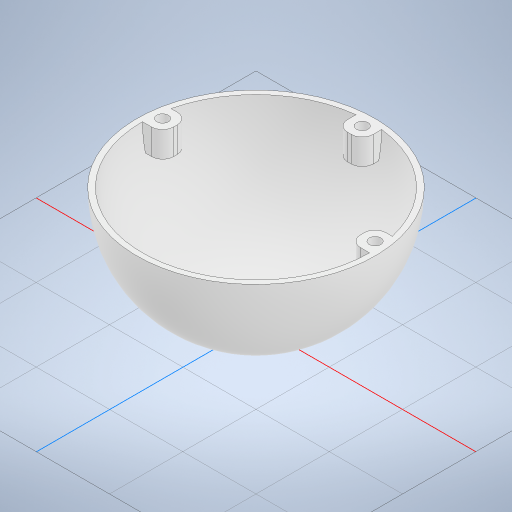
# Autodesk Inventor part: Kugel_part1_halbkugel
Saved by Autodesk Inventor 2023 (Build 270158000, 158)
## iProperties
Created: 2022-07-05
Part Number: Kugel_part1_halbkugel
Material: FormLabs Resin
Document SubType Name: Modeling
Designer: dennis
Density: 1.06 g/cm^3
Appearance: Smooth - White
Author: dennis
Autodesk Inventor part; units mm, degrees
ref_plane "YZ Plane" through (0, 0, 0) normal (1, 0, 0) x (0, 1, 0)
ref_plane "XZ Plane" through (0, 0, 0) normal (0, 1, 0) x (-1, 0, 0)
ref_plane "XY Plane" through (0, 0, 0) normal (0, 0, 1) x (1, 0, 0)
sketch "Skizze1" plane through (0, 0, 0) normal (0, 1, 0) x (-1, 0, 0)
  arc A0 (-32.5, 0) -> (32.5, 0) centre (0, 0) ccw
  line L0 (32.5, 0) -> (-32.5, 0)
  circle A1 centre (0, 0) radius 32.5
  line L1 (32.5, 0) -> (25.5, 0)
  line L2 (25.5, 0) -> (25.5, -7)
  line L3 (25.5, -7) -> (32.5, -7)
  line L4 (32.5, -7) -> (32.5, 0)
  line L5 (-32.5, 0) -> (-25.5, 0)
  line L6 (-25.5, 0) -> (-25.5, -7)
  line L7 (-25.5, -7) -> (-32.5, -7)
  line L8 (-32.5, -7) -> (-32.5, 0)
  line L9 (-3.5, -25.5) -> (3.5, -25.5)
  line L10 (3.5, -25.5) -> (3.5, -32.5)
  line L11 (3.5, -32.5) -> (-3.5, -32.5)
  line L12 (-3.5, -32.5) -> (-3.5, -25.5)
  line L13 (0, 0) -> (0, -32.5)
  circle A2 centre (29, -3.5) radius 1.6
  circle A3 centre (-29, -3.5) radius 1.6
  circle A4 centre (0, -29) radius 1.6
  point P0 (32.5, 0)
  point P1 (-31.7372, -7)
  point P2 (-25.5, 0)
  point P3 (-3.5, -32.311)
  point P4 (3.5, -32.311)
  point P5 (31.7372, -7)
  dimension "d0" = 65
  dimension "d2" = 65
  dimension "d3" = 7
  dimension "d4" = 7
  dimension "d5" = 7
  dimension "d6" = 7
  dimension "d20" = 7
  dimension "d21" = 7
  dimension "d22" = 32.5
  dimension "d23" = 3.2
  dimension "d24" = 3.2
  dimension "d25" = 3.2
  constraints: 28 end point, 6 parallel, 5 centre point, 4 horizontal, 3 perpendicular, 3 point on circle, 2 coincident, 1 point on line
  measures "d0" diameter of A0
  measures "d2" diameter of A1
  measures "d3" distance of L3.end L2.end
  measures "d4" distance of L2.end L1.end
  measures "d5" distance of L6.end L7.end
  measures "d6" distance of L5.end L6.end
  measures "d20" distance of L9.start L9.end
  measures "d21" distance of L11.end L9.start
  measures "d22" distance of L13.start L13.end
  measures "d23" diameter of A2
  measures "d24" diameter of A3
  measures "d25" diameter of A4
revolve "Umdrehung1" add sketch "Skizze1" angle 360 about axis through (-32.5, 0, 0) along (1, 0, 0) contours L0 L6 L7 A0 | L7 L6 L0 L13 L9 L12 A0 | A0 L3 L2 L0 | L12 L9 L13 A4 A0 | L0 L2 L3 A0 L10 L9 L13 | L13 A4 L9 L10 A0 | A4 L13 | L13 A4 | A2 | A3
extrude "Extrusion1" cut sketch "Skizze1" along normal up to surface contours L0 L6 L7 A0 | A1 L0 | L7 L6 L0 L13 L9 L12 A0 | A0 L3 L2 L0 | L12 L9 L13 A4 A0 | L0 L2 L3 A0 L10 L9 L13 | L13 A4 L9 L10 A0 | A4 L13 | L13 A4 | A2 | A3
shell "Wandung1" thickness 1.5 removed faces 1 at (-6.154, 0, 8.9157)
extrude "Extrusion2" add sketch "Skizze1" against normal blind 7 contours L0 L6 L7 A0 | A0 L3 L2 L0 | L12 L9 L13 A4 A0 | L13 A4 L9 L10 A0 | A4 L13 | L13 A4 | A2 | A3
delete faces "Fläche löschen1" heal yes whole lump no faces at (32.1325, -6.229, 0) (31.3606, -7, -6.2294) (32.4622, -2.3333, -1.5672) (31.3606, -6.2294, -7) (-1.9471, -2.3333, -32.4416) (-2.7229, -7, -31.8568) (3.5, -6.2291, -31.9413) (-3.5, -6.2291, -31.9413) (-32.4622, -2.3333, -1.5672) (-31.3606, -7, -6.2294) (-31.3606, -6.2294, -7) (-32.1325, -6.229, 0)
extrude "Extrusion3" cut sketch "Skizze1" against normal blind 5 contours A4 L13 | L13 A4 | A2 | A3
fillet "Rundung1" radius 3 6 edges at (3.5, -3.5, -25.5) (-3.5, -3.5, -25.5) (-25.5, -3.5, -7) (-25.5, -3.5, 0) (25.5, -3.5, 0) (25.5, -3.5, -7)
